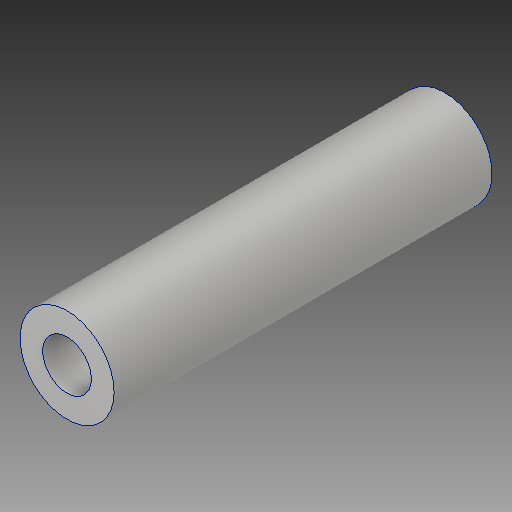
# Autodesk Inventor part: 2AM-17-P-4201 - tube shaft
Saved by Autodesk Inventor 2017 (Build 210142000, 142)
## iProperties
Created: 2017-12-27
Part Number: 2AM-17-P-4201 - tube shaft
Material: Aluminum 6061
Document SubType Name: Modeling
Designer: Micah
Density: 2.7 g/cm^3
Appearance: Aluminum - Flat
Mass: 12.6101 g
Surface Area: 32.4844 cm^2
Volume: 4.6704 cm^3
Author: Micah
Autodesk Inventor part; units mm, degrees
ref_plane "YZ Plane" through (0, 0, 0) normal (1, 0, 0) x (0, 1, 0)
ref_plane "XZ Plane" through (0, 0, 0) normal (0, 1, 0) x (-1, 0, 0)
ref_plane "XY Plane" through (0, 0, 0) normal (0, 0, 1) x (1, 0, 0)
sketch "Sketch1" plane through (0, 0, 0) normal (0, 0, 1) x (1, 0, 0)
  circle A0 centre (0, 0) radius 3.2766
  circle A1 centre (0, 0) radius 6.3246
  dimension "d0" = 50.8
  constraints: 2 centre point
extrude "Extrusion1" add sketch "Sketch1" along normal blind 50.8
body "Solid1"
